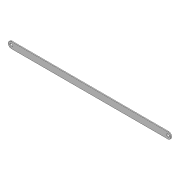
# Autodesk Inventor part: biela
Saved by Autodesk Inventor 2020 (Build 240168000, 168)
## iProperties
Created: 2022-05-07
Part Number: biela
Material: Generic
Document SubType Name: Modeling
Designer: leo
Density: 1 g/cm^3
Appearance: Default
Author: leo
Autodesk Inventor part; units mm, degrees
ref_plane "YZ Plane" through (0, 0, 0) normal (1, 0, 0) x (0, 1, 0)
ref_plane "XZ Plane" through (0, 0, 0) normal (0, 1, 0) x (-1, 0, 0)
ref_plane "XY Plane" through (0, 0, 0) normal (0, 0, 1) x (1, 0, 0)
sketch "Sketch1" plane through (0, 0, 0) normal (0, 0, 1) x (1, 0, 0)
  line L0 (0, 0) -> (556, 0) construction
  line L1 (0, -11) -> (556, -11)
  line L2 (556, 11) -> (0, 11)
  arc A0 (0, 11) -> (0, -11) centre (0, 0) ccw
  arc A1 (556, -11) -> (556, 11) centre (556, 0) ccw
  circle A2 centre (0, 0) radius 5
  circle A3 centre (556, 0) radius 5
  point P0 (278, 0)
  dimension "d0" = 556
  dimension "d1" = 10
  dimension "d2" = 22
  constraints: 8 end point, 4 centre point, 4 point on circle, 4 tangent, 2 coincident, 1 equal radius, 1 horizontal, 1 midpoint, 1 parallel
  measures "d0" distance of L0.start L0.end
  measures "d1" diameter of A2
  measures "d2" distance between parallel lines of L2 L1
extrude "Extrusion1" add sketch "Sketch1" along normal blind 3
body "Solid1"
